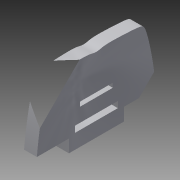
# Autodesk Inventor part: Interface_Left_Pannel
Saved by Autodesk Inventor 2016 (Build 200138000, 138)
## iProperties
Created: 2015-06-09
Part Number: Interface_Left_Pannel
Material: ABS Plastic
Document SubType Name: Modeling
Designer: Yann
Density: 1.06 g/cm^3
Appearance: Smooth - White
Author: Yann
Autodesk Inventor part; units mm, degrees
ref_plane "YZ Plane" through (0, 0, 0) normal (1, 0, 0) x (0, 1, 0)
ref_plane "XZ Plane" through (0, 0, 0) normal (0, 1, 0) x (-1, 0, 0)
ref_plane "XY Plane" through (0, 0, 0) normal (0, 0, 1) x (1, 0, 0)
sketch "Sketch1" plane through (0, 0, 0) normal (1, 0, 0) x (0, 1, 0)
  line L0 (-11.5, 1.2) -> (-11.5, 4.2) construction
  line L1 (11.5, 1.2) -> (11.5, 4.2) construction
  line L2 (0, 56.8321) -> (0, -15.3053) construction
  line L3 (-11.5, 2.7) -> (0, 2.7) construction
  line L4 (11.7, 1) -> (-11.7, 1)
  line L5 (-11.7, 1) -> (-11.7, 4.4)
  line L6 (-11.7, 4.4) -> (11.7, 4.4)
  line L7 (11.7, 4.4) -> (11.7, 1)
  line L8 (11.7, 1) -> (-11.7, 4.4) construction
  line L9 (-11.7, 1) -> (11.7, 4.4) construction
  line L10 (-8.75, 12.2) -> (-8.75, 14.2) construction
  line L11 (8.75, 12.2) -> (8.75, 14.2) construction
  line L12 (-8.75, 13.2) -> (8.75, 13.2) construction
  line L13 (8.95, 12) -> (-8.95, 12)
  line L14 (-8.95, 12) -> (-8.95, 14.4)
  line L15 (-8.95, 14.4) -> (8.95, 14.4)
  line L16 (8.95, 14.4) -> (8.95, 12)
  line L17 (8.95, 12) -> (-8.95, 14.4) construction
  line L18 (-8.95, 12) -> (8.95, 14.4) construction
  spline S0 degree 3 poles (0, 33.4863) (0.1363, 33.4863) (0.4006, 33.4933) (0.7102, 33.5178) (1.0034, 33.5518) (1.2244, 33.5856) (1.4837, 33.6328) (1.6778, 33.6734) (1.9519, 33.7353) (2.206, 33.7973) (2.5291, 33.876) (2.7703, 33.9323) (3.0216, 33.9864) (3.1959, 34.0215) (3.4716, 34.0725) (3.7687, 34.1211) (4.2651, 34.1883) (4.765, 34.2407) (5.4685, 34.294) (6.0941, 34.326) (6.9505, 34.3515) (7.6921, 34.3602) (8.8755, 34.3568) (10.1423, 34.3329) (11.8977, 34.2781) (13.2302, 34.2248) (14.5435, 34.1658) (15.4048, 34.1242) (16.4532, 34.0702) (17.2656, 34.0256) (18.2404, 33.9683) (18.9849, 33.9212) (19.8657, 33.8601) (20.5286, 33.8092) (21.3013, 33.7419) (21.8735, 33.6846) (22.5294, 33.6073) (23.0064, 33.5403) (23.5426, 33.4491) (23.9231, 33.37) (24.3377, 33.2635) (24.6209, 33.1729) (24.9192, 33.054) (25.1173, 32.9552) (25.3304, 32.8234) (25.4825, 32.7072) (25.6705, 32.5306) (25.826, 32.3538) (26.0357, 32.0643) (26.2161, 31.7693) (26.4569, 31.3049) (26.6607, 30.8521) (26.9823, 30.0385) (27.3257, 29.0379) (27.825, 27.3577) (28.2334, 25.8212) (28.6696, 24.0397) (28.9739, 22.7254) (29.3695, 20.9135) (29.6971, 19.3245) (30.117, 17.1531) (30.4593, 15.2636) (30.9755, 12.1876) (31.6613, 7.6456) (32.2185, 2.9449) (32.5, 0) knots 1.003531 1.003531 1.003531 1.003531 1.045161 1.08679 1.107605 1.149235 1.17005 1.21168 1.232495 1.29494 1.33657 1.399015 1.41983 1.461459 1.482274 1.544719 1.586349 1.669609 1.711239 1.794499 1.836128 1.919388 1.961018 2.085908 2.169168 2.294057 2.335687 2.418947 2.460577 2.543837 2.585466 2.668726 2.710356 2.793616 2.835246 2.918506 2.960135 3.043395 3.085025 3.168285 3.209915 3.293175 3.334804 3.418064 3.459694 3.542954 3.584584 3.667844 3.709473 3.792733 3.834363 3.917623 3.959253 4.084142 4.167402 4.292292 4.333922 4.417182 4.458811 4.542071 4.583701 4.666961 4.708591 4.83348 5 5 5 5 projected
  line L19 (-32.5, 0) -> (-15, 0)
  line L20 (-15, 0) -> (-15, -7)
  line L21 (-15, -7) -> (15, -7)
  line L22 (15, -7) -> (15, 0)
  line L23 (15, 0) -> (32.5, 0)
  spline S1 degree 3 poles (-32.5, 0) (-32.2185, 2.9449) (-31.6613, 7.6456) (-30.9755, 12.1876) (-30.4593, 15.2636) (-30.117, 17.1531) (-29.6971, 19.3245) (-29.3695, 20.9135) (-28.9739, 22.7254) (-28.6696, 24.0397) (-28.2334, 25.8212) (-27.825, 27.3577) (-27.3257, 29.0379) (-26.9823, 30.0385) (-26.6607, 30.8521) (-26.4569, 31.3049) (-26.2161, 31.7693) (-26.0357, 32.0643) (-25.826, 32.3538) (-25.6705, 32.5306) (-25.4825, 32.7072) (-25.3304, 32.8234) (-25.1173, 32.9552) (-24.9192, 33.054) (-24.6209, 33.1729) (-24.3377, 33.2635) (-23.9231, 33.37) (-23.5426, 33.4491) (-23.0064, 33.5403) (-22.5294, 33.6073) (-21.8735, 33.6846) (-21.3013, 33.7419) (-20.5286, 33.8092) (-19.8657, 33.8601) (-18.9849, 33.9212) (-18.2404, 33.9683) (-17.2656, 34.0256) (-16.4532, 34.0702) (-15.4048, 34.1242) (-14.5435, 34.1658) (-13.2302, 34.2248) (-11.8977, 34.2781) (-10.1423, 34.3329) (-8.8755, 34.3568) (-7.6921, 34.3602) (-6.9505, 34.3515) (-6.0941, 34.326) (-5.4685, 34.294) (-4.765, 34.2407) (-4.2651, 34.1883) (-3.7687, 34.1211) (-3.4716, 34.0725) (-3.1959, 34.0215) (-3.0216, 33.9864) (-2.7703, 33.9323) (-2.5291, 33.876) (-2.206, 33.7973) (-1.9519, 33.7353) (-1.6778, 33.6734) (-1.4837, 33.6328) (-1.2244, 33.5856) (-1.0034, 33.5518) (-0.7102, 33.5178) (-0.4006, 33.4933) (-0.1363, 33.4863) (0, 33.4863) knots 1.003531 1.003531 1.003531 1.003531 1.17005 1.29494 1.33657 1.41983 1.461459 1.544719 1.586349 1.669609 1.711239 1.836128 1.919388 2.044278 2.085908 2.169168 2.210797 2.294057 2.335687 2.418947 2.460577 2.543837 2.585466 2.668726 2.710356 2.793616 2.835246 2.918506 2.960135 3.043395 3.085025 3.168285 3.209915 3.293175 3.334804 3.418064 3.459694 3.542954 3.584584 3.667844 3.709473 3.834363 3.917623 4.042513 4.084142 4.167402 4.209032 4.292292 4.333922 4.417182 4.458811 4.521256 4.542071 4.583701 4.604516 4.666961 4.708591 4.771036 4.791851 4.83348 4.854295 4.895925 4.91674 4.95837 5 5 5 5 projected
  point P0 (0, 0)
  point P1 (0, 33.4863)
  point P2 (0, 13.2)
  dimension "d0" = 0.2
  dimension "d1" = 0.2
  dimension "d2" = 0.2
  dimension "d3" = 0.2
  dimension "d6" = 30
  dimension "d7" = 7
  constraints: 38 end point, 8 midpoint, 7 perpendicular, 4 horizontal, 4 parallel, 2 point on line, 1 other
  measures "d0" distance between parallel lines of L5 L0
  measures "d1" distance from line of L0.end L6
  measures "d2" distance from line of L12.start L14
  measures "d3" distance from line of L10.end L15
  measures "d6" distance between parallel lines of L22 L20
  measures "d7" distance between parallel lines of L19 L21
extrude "Extrusion1" add sketch "Sketch1" against normal blind 7
fillet "Fillet1" radius 4 2 edges at (-7, 15, -3.5) (-7, -15, -3.5)
equation "\"d2\" = d1"
equation "\"d3\" = d2"
equation "\"d7\" = Heatsink_Thickness"
equation "\"d4\" = Interface_Thickness"
equation "\"Heatsink_Thickness\" = 7"
equation "\"Interface_Thickness\" = 7"
equation "\"Heatsink_Width\" = 65"
equation "\"Cover_Thickness\" = 2"
equation "\"PowerPCB_Minus_Height\" = 1.2"
equation "\"PowerPCB_Thickness\" = 3"
equation "\"PowerPCB_Plus_Height\" = 8"
equation "\"LogicPCB_Width\" = 55"
equation "\"LogicPCB_Thickness\" = 2"
equation "\"LogicPCB_Plus_Height\" = 8"
equation "\"HostPCB_Thickness\" = 1.2"
equation "\"HostPCB_Plus_Height\" = 8"
body "Solid1"
